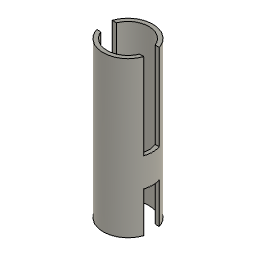
CrokinoleHolder (Autodesk Fusion 360 design; units mm, degrees)
Autodesk Fusion 360 part; units mm, degrees
sketch "Sketch1" plane through (0, 0, 0) normal (0, 0, 1) x (1, 0, 0)
  circle A0 centre (0, 0) radius 19
  circle A1 centre (0, 0) radius 16
  dimension "d6" = 38
  dimension "d7" = 32
  constraint coincident A0.centre A1.centre
  constraint concentric A0 A1
  measures "d6" diameter of A0
  measures "d7" diameter of A1
extrude "Extrude1" add sketch "Sketch1" along normal blind 119
sketch "Sketch2" plane through (0, 0, 0) normal (0, 0, 1) x (1, 0, 0)
  line L0 (32, 6) -> (-32, 6)
  line L1 (-32, 6) -> (-32, -6)
  line L2 (-32, -6) -> (32, -6)
  line L3 (32, -6) -> (32, 6)
  line L4 (32, 6) -> (-32, -6) construction
  line L5 (-32, 6) -> (32, -6) construction
  dimension "d10" = 64
  dimension "d11" = 12
  constraint horizontal L0
  constraint perpendicular L0 L1
  constraint parallel L0 L2
  constraint parallel L1 L3
  constraint coincident L4 origin
  constraint coincident L5 origin
  measures "d10" distance of L1.end L2.end
  measures "d11" distance of L0.end L1.end
extrude "Extrude2" cut sketch "Sketch2" along normal blind 31
ref_plane "WorkPlane1" through (0, 0, 119) normal (0, 0, 1) x (1, 0, 0)
sketch "Sketch3" plane through (0, 0, 119) normal (0, 0, 1) x (1, 0, 0)
  line L0 (32, 6) -> (-32, 6)
  line L1 (-32, 6) -> (-32, -6)
  line L2 (-32, -6) -> (32, -6)
  line L3 (32, -6) -> (32, 6)
  line L4 (32, 6) -> (-32, -6) construction
  line L5 (-32, 6) -> (32, -6) construction
  dimension "d15" = 64
  dimension "d16" = 12
  constraint horizontal L0
  constraint perpendicular L0 L1
  constraint parallel L0 L2
  constraint parallel L1 L3
  constraint coincident L4 origin
  constraint coincident L5 origin
  measures "d15" distance of L1.end L2.end
  measures "d16" distance of L0.end L1.end
extrude "Extrude3" cut sketch "Sketch3" against normal blind 66
equation "discDia = 32 mm"
equation "discHeight = 11 mm"
equation "gutterRim = 12 mm"
equation "gutterDepth = 31 mm"
equation "wall = 3 mm"
equation "d6 = discDia + wall * 2"
equation "d7 = discDia"
equation "d8 = gutterDepth + discAreaHeight"
equation "d10 = discDia * 2"
equation "d11 = gutterRim"
equation "d12 = gutterDepth"
equation "d14 = gutterDepth + discAreaHeight"
equation "d15 = discDia * 2"
equation "d16 = gutterRim"
equation "d17 = -discAreaHeight + 2 * discHeight"
equation "discAreaHeight = discHeight * 8"
